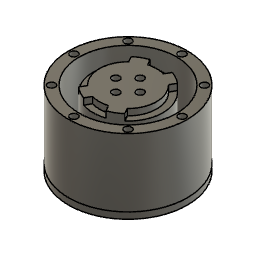
ruedaSilicona v13 (Autodesk Fusion 360 design; units mm, degrees)
Autodesk Fusion 360 part; units mm, degrees
sketch "Boceto1" plane through (0, 0, 0) normal (0, 1, 0) x (1, 0, 0)
  circle A0 centre (0, 0) radius 16.5
  circle A1 centre (0, 0) radius 23
  circle A2 centre (0, 0) radius 28
  line L0 (0, 0) -> (0, -23) construction
  line L1 (0, -23) -> (0, -28) construction
  circle A3 centre (0, -25.5) radius 1.75
  circle A4 centre (25.5, 0) radius 1.75
  circle A5 centre (0, 25.5) radius 1.75
  circle A6 centre (-25.5, 0) radius 1.75
  circle A7 centre (0, 0) radius 1.5 construction
  line L2 (0, 0) -> (-16.5, 0) construction
  circle A8 centre (0, 0) radius 11.5 construction
  line L3 (0, 0) -> (-5.75, -9.959292) construction
  line L4 (0, 0) -> (-11.5, 0) construction
  line L5 (-5.75, -9.959292) -> (-8.25, -14.289419) construction
  line L6 (-2.70102, -11.178304) -> (-5.273796, -15.634483)
  line L7 (-8.330185, -7.928304) -> (-10.902962, -12.384483)
  line L8 (8.330185, -7.928304) -> (10.902962, -12.384483)
  line L9 (2.70102, -11.178304) -> (5.273796, -15.634483)
  line L10 (8.330185, 7.928304) -> (10.902962, 12.384483)
  line L11 (2.70102, 11.178304) -> (5.273796, 15.634483)
  line L12 (-2.70102, 11.178304) -> (-5.273796, 15.634483)
  line L13 (-8.330185, 7.928304) -> (-10.902962, 12.384483)
  circle A9 centre (0, 0) radius 13.5
  line L14 (0, 0) -> (0, 5.75) construction
  circle A10 centre (0, 5.75) radius 1.75
  circle A11 centre (-5.75, 0) radius 1.75
  circle A12 centre (0, -5.75) radius 1.75
  circle A13 centre (5.75, 0) radius 1.75
  circle A14 centre (18.031223, -18.031223) radius 1.75
  circle A15 centre (25.5, 0) radius 1.75
  circle A16 centre (18.031223, 18.031223) radius 1.75
  circle A17 centre (0, 25.5) radius 1.75
  circle A18 centre (-18.031223, 18.031223) radius 1.75
  circle A19 centre (-25.5, 0) radius 1.75
  circle A20 centre (-18.031223, -18.031223) radius 1.75
  dimension "d1" = 33
  dimension "d2" = 46
  dimension "d3" = 56
  dimension "d18" = 3.5
  dimension "d20" = 360
  dimension "d21" = 3
  dimension "d24" = 23
  dimension "d25" = 60
  dimension "d26" = 3.25
  dimension "d27" = 2
  dimension "d41" = 5.75
  dimension "d42" = 3.5
  dimension "d44" = 360
  dimension "d46" = 360
  constraint coincident A0.centre A1.centre
  constraint concentric A0 A1
  constraint coincident A1 L0.end
  constraint vertical L0
  constraint coincident A2 L1.end
  constraint parallel L0 L1
  constraint midpoint L1 A3.centre
  constraint horizontal L2
  constraint concentric A0 A8
  constraint horizontal L4
  constraint parallel L3 L5
  constraint parallel L5 L6
  constraint coincident A8 L4.end
  constraint coincident A0 L2.end
  constraint perpendicular L4 L14
  constraint coincident L14.end A10.centre
  measures "d1" diameter of A0
  measures "d2" diameter of A1
  measures "d3" diameter of A2
  measures "d18" diameter of A3
  measures "d21" diameter of A7
  measures "d24" diameter of A8
  measures "d25" angle of L3 L4
  measures "d26" distance of L5 L6
  measures "d41" distance of A0.centre L14.end
  measures "d42" diameter of A10
extrude "Extruir1" add sketch "Boceto1" along normal blind 32 makes body 1 at (16.479489, 10.666667, 0.822457) makes body 2 at (27.965194, 21.333333, 1.395685)
extrude "Extruir5" cut sketch "Boceto1" along normal blind 3 contours A0 L8 L10 A9 | A0 L11 L12 A9 | A0 L6 L9 A9 | A0 L7 L13 A9 picked at (10.936485, 10.943401) picked at (0, 15.476723) picked at (0, -15.476723) picked at (-15.433023, 1.104238) bodies 1
extrude "Extruir6" cut sketch "Boceto1" against normal blind 3 from surface at 32 contours A0 L8 L10 A9 | A0 L11 L12 A9 | A0 L6 L9 A9 | A0 L7 L13 A9 picked at (10.936485, 10.943401) picked at (0, 15.476723) picked at (0, -15.476723) picked at (-15.433023, 1.104238) bodies 1
extrude "Extruir2" add sketch "Boceto1" against normal blind 3 separate body contours A0 L8 L10 A9 | A0 L10 L11 A9 | A0 L8 L9 A9 | A0 L11 L12 A9 | A9 | A0 L6 L9 A9 | A0 L12 L13 A9 | A0 L6 L7 A9 | A0 L7 L13 A9 | A1 | A2 picked at (10.936485, 10.943401) picked at (7.737993, 13.402597) picked at (7.737993, -13.402597) picked at (0, 15.476723) picked at (5.659098, -5.826142) picked at (0, -15.476723) picked at (-7.737993, 13.402597) picked at (-7.737993, -13.402597) picked at (-15.433023, 1.104238) picked at (-11.671979, 17.204699) picked at (-14.082794, -21.129607) makes body 3
ref_plane "PlanoDeObra2" through (14.289419, 19.767485, -8.25) normal (0.866025, 0, -0.5) x (0.5, 0, 0.866025)
sketch "Boceto3" plane through (14.289419, 21.564529, -8.25) normal (0.866025, 0, -0.5) x (0.5, 0, 0.866025)
  line L0 (16.176758, -7.435471) -> (16.176758, -10.435471)
  line L1 (16.176758, -10.435471) -> (16.5, -10.435471)
  line L2 (16.176758, -10.435471) -> (16.176758, -7.435471)
  line L3 (16.176758, -7.435471) -> (10.902962, -7.435471)
  line L4 (10.902962, -7.435471) -> (10.902962, -10.435471)
  line L5 (5.273796, -10.435471) -> (10.902962, -10.435471)
  line L6 (5.273796, -10.435471) -> (5.273796, -7.435471)
  line L7 (5.273796, -7.435471) -> (-16.176758, -7.435471)
  line L8 (-16.176758, -7.435471) -> (-16.176758, -10.435471)
  line L9 (-16.5, -10.435471) -> (-16.176758, -10.435471)
  line L10 (-16.176758, -10.435471) -> (-16.176758, -7.435471)
  line L11 (-10.902962, -7.435471) -> (-16.176758, -7.435471)
  line L12 (-10.902962, -7.435471) -> (-10.902962, -10.435471)
  line L13 (-10.902962, -10.435471) -> (-5.273796, -10.435471)
  line L14 (-5.273796, -10.435471) -> (-5.273796, -7.435471)
  line L15 (16.176758, -7.435471) -> (-5.273796, -7.435471)
  line L16 (16.176758, 21.564529) -> (16.176758, 18.564529)
  line L17 (-5.273796, 18.564529) -> (16.176758, 18.564529)
  line L18 (-5.273796, 18.564529) -> (-5.273796, 21.564529)
  line L19 (-10.902962, 21.564529) -> (-5.273796, 21.564529)
  line L20 (-10.902962, 21.564529) -> (-10.902962, 18.564529)
  line L21 (-16.176758, 18.564529) -> (-10.902962, 18.564529)
  line L22 (-16.176758, 18.564529) -> (-16.176758, 21.564529)
  line L23 (-16.5, 21.564529) -> (-16.176758, 21.564529)
  line L24 (-16.176758, 21.564529) -> (-16.176758, 18.564529)
  line L25 (-16.176758, 18.564529) -> (5.273796, 18.564529)
  line L26 (5.273796, 18.564529) -> (5.273796, 21.564529)
  line L27 (5.273796, 21.564529) -> (10.902962, 21.564529)
  line L28 (10.902962, 21.564529) -> (10.902962, 18.564529)
  line L29 (10.902962, 18.564529) -> (16.176758, 18.564529)
  line L30 (16.176758, 18.564529) -> (16.176758, 21.564529)
  line L31 (16.176758, 21.564529) -> (16.5, 21.564529)
  line L32 (0, 18.564529) -> (0, -7.435474) construction
  circle A0 centre (0, 5.564527) radius 3
  dimension "d34" = 6
  constraint coincident origin L32
  constraint parallel L24 L32
  measures "d34" diameter of A0
extrude "Extruir7" cut sketch "Boceto3" against normal blind 3 contours A0 picked at (-0.5, 6.560249) bodies 1
mirror "Simetría1" about plane through (0, 0, 0) normal (1, 0, 0) of "Extruir7"
mirror "Simetría2" about plane through (0, 0, 0) normal (0, 0, 1) of "Extruir7", "Simetría1"
named bodies: "centroMolde", "bordeMolde", "pisoMolde"
